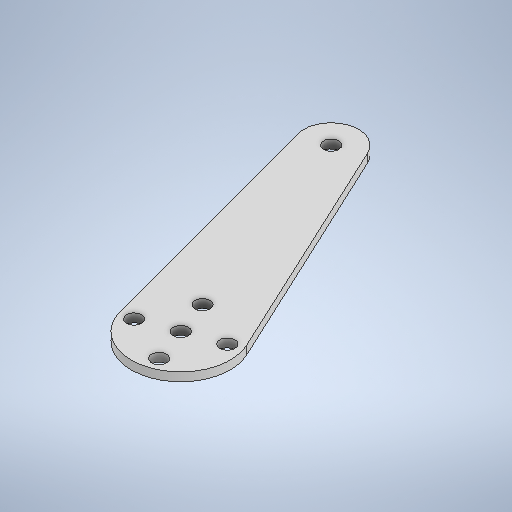
# Autodesk Inventor part: A1P1
Saved by Autodesk Inventor 2025.2 (Build 292293000, 293)
## iProperties
Created: 2025-05-21
Part Number: A1P1
Material: Generic
Document SubType Name: Sheet Metal
Designer: Admin
Density: 1 g/cm^3
Sheet Metal Rule: Default
Appearance: Default
Author: Admin
Autodesk Inventor part; units mm, degrees
ref_plane "YZ Plane" through (0, 0, 0) normal (1, 0, 0) x (0, 1, 0)
ref_plane "XZ Plane" through (0, 0, 0) normal (0, 1, 0) x (-1, 0, 0)
ref_plane "XY Plane" through (0, 0, 0) normal (0, 0, 1) x (1, 0, 0)
sketch "Sketch1" plane through (0, 0, 0) normal (0, 1, 0) x (-1, 0, 0)
  arc A0 (9.4829, 2.5433) -> (-8.8962, -4.1533) centre (0, 0) ccw
  line L0 (9.4829, 2.5433) -> (22.3854, -45.5658)
  line L1 (-8.8962, -4.1533) -> (12.1747, -49.2862)
  arc A1 (12.1747, -49.2862) -> (22.3854, -45.5658) centre (17.1171, -46.9788) ccw
  dimension "d0" = 19.636
  dimension "d3" = 5.4545
  dimension "d18" = 50
  constraints: 4 end point, 4 point on circle, 4 tangent, 2 centre point, 1 coincident
  measures "d0" diameter of A0
  measures "d3" radius of A1
  measures "d18" distance of point (0, 0) A1.centre
extrude "Extrusion1" add sketch "Sketch1" along normal blind 1.7
sketch "Sketch2" plane through (0, 1.7, 0) normal (0, 1, 0) x (1, 0, 0)
  arc A0 (-12.1747, 49.2862) -> (-22.3854, 45.5658) centre (-17.1171, 46.9788) ccw projected
  arc A1 (-9.4829, -2.5433) -> (8.8962, 4.1533) centre (0, 0) ccw projected
  circle A2 centre (0, 0) radius 1.5
  circle A3 centre (-17.1171, 46.9788) radius 1.5
  circle A4 centre (6.7831, 2.4715) radius 1.5
  circle A5 centre (-6.7831, -2.4715) radius 1.5
  circle A6 centre (-2.4714, 6.7828) radius 1.5
  circle A7 centre (2.4714, -6.7828) radius 1.5
  line L0 (-17.1171, 46.9788) -> (0, 0) construction
  line L1 (-17.1171, 46.9788) -> (-2.4714, 6.7828) construction
  line L2 (0, 0) -> (2.4714, -6.7828) construction
  line L3 (-6.7831, -2.4715) -> (0, 0) construction
  line L4 (0, 0) -> (6.7831, 2.4715) construction
  dimension "d4" = 3
  dimension "d5" = 3
  dimension "d6" = 3
  dimension "d7" = 3
  dimension "d12" = 3
  dimension "d13" = 3
  dimension "d19" = 7.219
  dimension "d20" = 7.2193
  dimension "d21" = 7.2193
  dimension "d22" = 7.219
  constraints: 10 end point, 6 centre point, 3 collinear, 2 coincident, 1 perpendicular
  measures "d4" diameter of A2
  measures "d5" diameter of A3
  measures "d6" diameter of A4
  measures "d7" diameter of A5
  measures "d12" diameter of A6
  measures "d13" diameter of A7
  measures "d19" distance of L0.end L2.end
  measures "d20" distance of L0.end L4.end
  measures "d21" distance of L3.start L0.end
  measures "d22" distance of point (0, 0) L1.end
extrude "Extrusion2" cut sketch "Sketch2" against normal blind 1.7
equation "\"BendRadius\" = Thickness"
equation "\"BendReliefWidth\" = Thickness"
equation "\"BendReliefDepth\" = 0.5 * Thickness"
equation "\"CornerReliefSize\" = 4 * Thickness"
equation "\"MinimumRemnant\" = 2 * Thickness"
equation "\"TransitionRadius\" = BendRadius"
equation "\"JacobiRadiusSize\" = BendRadius"
equation "\"GapSize\" = Thickness"
equation "\"Thickness\" = 3.048"
body "Solid1"
